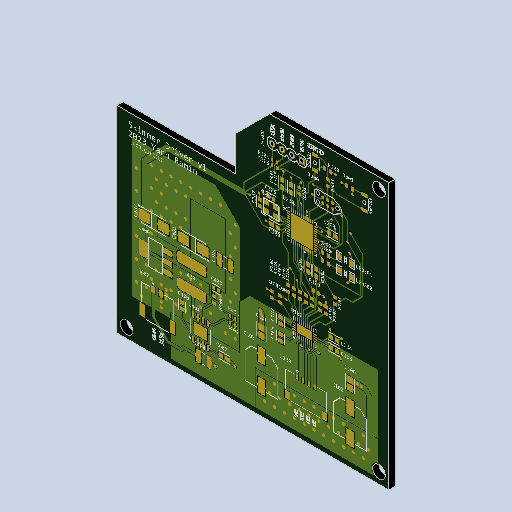
# Autodesk Inventor part: skimmer_swabbie_v1_BOARD
Saved by Autodesk Inventor 2023.2 (Build 272271000, 271)
## iProperties
Created: 2023-03-08
Part Number: skimmer_swabbie_v1_BOARD
Material: Generic
Document SubType Name: Modeling
Designer: atrus
Density: 1 g/cm^3
Appearance: BoardColor
Author: atrus
Autodesk Inventor part; units mm, degrees
ref_plane "YZ Plane" through (0, 0, 0) normal (1, 0, 0) x (0, 1, 0)
ref_plane "XZ Plane" through (0, 0, 0) normal (0, 1, 0) x (-1, 0, 0)
ref_plane "BoardFrontPlane" through (0, 0, 0) normal (0, 0, 1) x (1, 0, 0)
sketch "Sketch1" plane through (0, 0, 0) normal (0, 0, 1) x (1, 0, 0)
  line L0 (43.18, 34.29) -> (43.18, 85.09)
  line L1 (43.18, 85.09) -> (73.66, 85.09)
  line L2 (73.66, 85.09) -> (73.66, 93.98)
  line L3 (73.66, 93.98) -> (82.55, 102.87)
  line L4 (82.55, 102.87) -> (113.284, 102.87)
  line L5 (113.284, 102.87) -> (113.284, 34.29)
  line L6 (113.284, 34.29) -> (43.18, 34.29)
  constraints: 14 end point
extrude "BoardOutline" add sketch "Sketch1" along normal blind 1.6194
sketch "img_Top" plane through (0, 0, 1.6194) normal (0, 0, 1) x (1, 0, 0)
  line L0 (43.18, 102.87) -> (113.284, 102.87) construction
  line L1 (113.284, 102.87) -> (113.284, 34.29) construction
  line L2 (113.284, 34.29) -> (43.18, 34.29) construction
  line L3 (43.18, 34.29) -> (43.18, 102.87) construction
  constraints: 2 other
decal "Decal_Top"
sketch "img_Bottom" plane through (0, 0, -1.6194) normal (0, 0, -1) x (1, 0, 0)
  line L0 (43.18, -34.29) -> (113.284, -34.29) construction
  line L1 (113.284, -34.29) -> (113.284, -102.87) construction
  line L2 (113.284, -102.87) -> (43.18, -102.87) construction
  line L3 (43.18, -102.87) -> (43.18, -34.29) construction
  constraints: 2 other
decal "Decal_Bottom"
sketch "Sketch4" plane through (0, 0, 1.6194) normal (0, 0, 1) x (1, 0, 0)
  point P0 (94.234, 97.79)
hole "SW301-H1" at (94.234, 97.79, 1.6194) direction (0, 0, -1) diameter 0.85 end through all
sketch "Sketch5" plane through (0, 0, 1.6194) normal (0, 0, 1) x (1, 0, 0)
  point P0 (106.934, 95.25)
hole "SW300-H1" at (106.934, 95.25, 1.6194) direction (0, 0, -1) diameter 0.85 end through all
sketch "Sketch6" plane through (0, 0, 1.6194) normal (0, 0, 1) x (1, 0, 0)
  point P0 (45.72, 36.83)
hole "Free-MNT+4" at (45.72, 36.83, 1.6194) direction (0, 0, -1) diameter 3.2512 end through all
sketch "Sketch7" plane through (0, 0, 1.6194) normal (0, 0, 1) x (1, 0, 0)
  point P0 (110.744, 37.084)
hole "Free-MNT+3" at (110.744, 37.084, 1.6194) direction (0, 0, -1) diameter 3.2512 end through all
sketch "Sketch8" plane through (0, 0, 1.6194) normal (0, 0, 1) x (1, 0, 0)
  point P0 (110.744, 100.076)
hole "Free-MNT+2" at (110.744, 100.076, 1.6194) direction (0, 0, -1) diameter 3.2512 end through all
sketch "Sketch9" plane through (0, 0, 1.6194) normal (0, 0, 1) x (1, 0, 0)
  point P0 (90.805, 96.52)
hole "JP300-1" at (90.805, 96.52, 1.6194) direction (0, 0, -1) diameter 1.016 end through all
sketch "Sketch10" plane through (0, 0, 1.6194) normal (0, 0, 1) x (1, 0, 0)
  point P0 (88.265, 96.52)
hole "JP300-2" at (88.265, 96.52, 1.6194) direction (0, 0, -1) diameter 1.016 end through all
sketch "Sketch11" plane through (0, 0, 1.6194) normal (0, 0, 1) x (1, 0, 0)
  point P0 (85.725, 96.52)
hole "JP300-3" at (85.725, 96.52, 1.6194) direction (0, 0, -1) diameter 1.016 end through all
sketch "Sketch12" plane through (0, 0, 1.6194) normal (0, 0, 1) x (1, 0, 0)
  point P0 (83.185, 96.52)
hole "JP300-4" at (83.185, 96.52, 1.6194) direction (0, 0, -1) diameter 1.016 end through all
sketch "Sketch13" plane through (0, 0, 1.6194) normal (0, 0, 1) x (1, 0, 0)
  point P0 (94.996, 91.44)
hole "J300-_OMJMIDLA" at (94.996, 91.44, 1.6194) direction (0, 0, -1) diameter 0.9 end through all
sketch "Sketch14" plane through (0, 0, 1.6194) normal (0, 0, 1) x (1, 0, 0)
  point P0 (94.996, 89.408)
hole "J300-_YAKUTFXJ" at (94.996, 89.408, 1.6194) direction (0, 0, -1) diameter 0.9 end through all
sketch "Sketch15" plane through (0, 0, 1.6194) normal (0, 0, 1) x (1, 0, 0)
  point P0 (100.076, 90.424)
hole "J300-_MBXSYRVB" at (100.076, 90.424, 1.6194) direction (0, 0, -1) diameter 0.9 end through all
body "Solid1"
